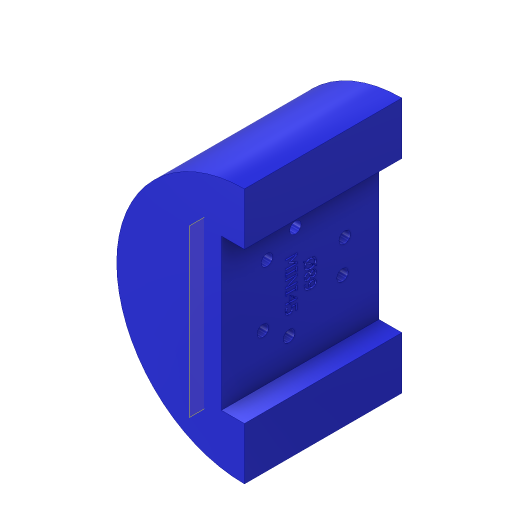
# Autodesk Inventor part: MINI45NewShell89_A
Saved by Autodesk Inventor 2023 (Build 270158000, 158)
## iProperties
Created: 2016-07-01
Part Number: MINI45NewShell89_A
Material: ABS Plastic
Document SubType Name: Modeling
Designer: Administrateur
Density: 1.06 g/cm^3
Appearance: Blue - Wall Paint - Glossy
Author: Administrateur
Autodesk Inventor part; units mm, degrees
ref_plane "XZ Plane" through (0, 0, 0) normal (0, 1, 0) x (-1, 0, 0)
sketch "Sketch1" plane through (0, 0, 0) normal (0, 0, 1) x (1, 0, 0)
  arc A0 (0, 38.9636) -> (0, -38.9636) centre (0, 0) ccw
  line L0 (0, 38.9636) -> (0, 23)
  line L1 (0, 23) -> (-7, 23)
  line L2 (-7, 23) -> (-7, 0)
  line L3 (-46.5484, 0) -> (26.4312, 0) construction
  line L4 (0, -38.9636) -> (0, -23)
  line L5 (0, -23) -> (-7, -23)
  line L6 (-7, -23) -> (-7, 0)
  dimension "d2" = 38.9636
  dimension "d3" = 46
  dimension "d4" = 7
  dimension "d27" = 23
  dimension "d28" = 15.9636
  constraints: 14 end point, 2 horizontal, 2 point on circle, 2 symmetric about line, 1 centre point, 1 coincident, 1 perpendicular, 1 vertical
  measures "d2" radius of A0
  measures "d3" distance between parallel lines of L5 L1
  measures "d4" distance of L0.end L1.end
  measures "d27" distance of L1.end L2.end
  measures "d28" distance of L0.start L0.end
extrude "Extrusion1" add sketch "Sketch1" along normal blind 48
sketch "Sketch2" plane through (-7, -23, 0) normal (1, 0, 0) x (0, 0, -1)
  line L0 (-24, 23) -> (-48, 23) construction
  line L1 (-48, 61.9636) -> (-48, -15.9636) construction
  line L2 (0, 61.9636) -> (-48, 61.9636) construction
  line L3 (-24, 61.9636) -> (-24, -15.9636) construction
  line L4 (0, -15.9636) -> (-48, -15.9636) construction
  line L5 (-24, 23) -> (-34.1427, 32.7947) construction
  circle A0 centre (-24, 23) radius 14.1 construction
  line L6 (-24, 23) -> (-25.4739, 37.0228) construction
  line L7 (-24, 23) -> (-27.4111, 9.3188) construction
  line L8 (-24, 23) -> (-35.4071, 14.7122) construction
  line L9 (-24, 23) -> (-10.4462, 26.8865) construction
  line L10 (-24, 23) -> (-11.119, 17.265) construction
  point P0 (0, 23)
  dimension "d32" = 28.2
  dimension "d34" = 40
  dimension "d37" = 360
  dimension "d39" = 84
  constraints: 16 end point, 11 coincident, 4 midpoint, 2 point on circle, 1 centre point, 17 other
  measures "d32" diameter of A0
  measures "d34" angle of L5 L6
  measures "d39" angle of L0 L6
hole "Hole1" at (-7, 14.0228, 25.4739) at (-7, 9.7947, 34.1427) at (-7, -8.2878, 35.4071) at (-7, -13.6812, 27.4111) at (-7, -5.735, 11.119) at (-7, 3.8865, 10.4462) direction (-1, 0, 0) diameter 3.5 end through all
ref_plane "Work Plane1" through (-38.9636, 0, 0) normal (1, 0, 0) x (0, 1, 0)
ref_plane "Work Plane2" through (-10, 0, 0) normal (1, 0, 0) x (0, 1, 0)
ref_plane "Work Plane3" through (-12.3, -23, 0) normal (1, 0, 0) x (0, 0, -1)
sketch "Sketch4" plane through (-12.3, -23, 0) normal (1, 0, 0) x (0, 0, -1)
  line L0 (0, 61.9636) -> (0, -15.9636) projected
  line L1 (0, -15.9636) -> (-48, -15.9636) projected
  line L2 (-48, 61.9636) -> (-48, -15.9636) projected
  line L3 (0, 61.9636) -> (-48, 61.9636) projected
  circle A0 centre (-25.4739, 37.0228) radius 1.75 projected
  circle A1 centre (-34.1427, 32.7947) radius 1.75 projected
  circle A2 centre (-35.4071, 14.7122) radius 1.75 projected
  circle A3 centre (-27.4111, 9.3188) radius 1.75 projected
  circle A4 centre (-11.119, 17.265) radius 1.75 projected
  circle A5 centre (-10.4462, 26.8865) radius 1.75 projected
  point P0 (0, 23)
  point P1 (-11.119, 19.015)
  point P2 (-35.4071, 16.4622)
  point P3 (-25.4739, 38.7728)
  point P4 (-34.1427, 34.5447)
  point P5 (-27.4111, 11.0688)
  point P6 (-10.4462, 28.6365)
  constraints: 6 coincident, 6 vertical alignment, 6 other
hole "Hole3" at (-12.3, 14.0228, 25.4739) at (-12.3, 9.7947, 34.1427) at (-12.3, -8.2878, 35.4071) at (-12.3, -13.6812, 27.4111) at (-12.3, -5.735, 11.119) at (-12.3, 3.8865, 10.4462) direction (-1, 0, 0) diameter 6.5 end through all
sketch "Sketch7" plane through (-7, -23, 0) normal (1, 0, 0) x (0, 0, -1)
  line L0 (-18.9668, 30.4561) -> (-18.9668, 14.6891) construction
  line L1 (-18.9668, 14.6891) -> (-28.3826, 14.6891) construction
  line L2 (-28.3826, 14.6891) -> (-28.3826, 30.4561) construction
  line L3 (-28.3826, 30.4561) -> (-18.9668, 30.4561) construction
  spline S0 degree 2 poles (-20.9323, 23.6518) (-21.8002, 23.6518) (-22.7561, 24.497) (-22.7561, 25.2004) knots 0 0 0 1 2 2 2
  spline S1 degree 2 poles (-22.7561, 25.2004) (-22.7561, 25.4585) (-22.6199, 25.9038) (-22.4951, 26.0825) knots 0 0 0 1 2 2 2
  line L4 (-22.4951, 26.0825) -> (-22.9546, 26.3945)
  line L5 (-22.9546, 26.3945) -> (-22.9546, 26.7405)
  line L6 (-22.9546, 26.7405) -> (-22.3023, 26.2981)
  spline S2 degree 2 poles (-22.3023, 26.2981) (-22.0697, 26.5079) (-21.3833, 26.7462) (-20.9323, 26.7462) knots 0 0 0 1 2 2 2
  spline S3 degree 2 poles (-20.9323, 26.7462) (-20.0672, 26.7462) (-19.1086, 25.8981) (-19.1086, 25.2004) knots 0 0 0 1 2 2 2
  spline S4 degree 2 poles (-19.1086, 25.2004) (-19.1086, 24.931) (-19.239, 24.5112) (-19.3667, 24.324) knots 0 0 0 1 2 2 2
  line L7 (-19.3667, 24.324) -> (-18.9668, 24.0545)
  line L8 (-18.9668, 24.0545) -> (-18.9668, 23.7057)
  line L9 (-18.9668, 23.7057) -> (-19.5567, 24.1084)
  spline S5 degree 2 poles (-19.5567, 24.1084) (-19.7893, 23.8929) (-20.4643, 23.6518) (-20.9323, 23.6518) knots 0 0 0 1 2 2 2
  spline S6 degree 2 poles (-20.9323, 24.1311) (-20.609, 24.1311) (-20.1013, 24.2616) (-19.9339, 24.3694) knots 0 0 0 1 2 2 2
  line L10 (-19.9339, 24.3694) -> (-22.1377, 25.8442)
  spline S7 degree 2 poles (-22.1377, 25.8442) (-22.2455, 25.7109) (-22.3533, 25.4103) (-22.3533, 25.1976) knots 0 0 0 1 2 2 2
  spline S8 degree 2 poles (-22.3533, 25.1976) (-22.3533, 24.7126) (-21.6215, 24.1311) (-20.9323, 24.1311) knots 0 0 0 1 2 2 2
  spline S9 degree 2 poles (-19.7212, 24.5622) (-19.6163, 24.6842) (-19.5113, 25.0047) (-19.5113, 25.1976) knots 0 0 0 1 2 2 2
  spline S10 degree 2 poles (-19.5113, 25.1976) (-19.5113, 25.6854) (-20.2346, 26.2669) (-20.9323, 26.2669) knots 0 0 0 1 2 2 2
  spline S11 degree 2 poles (-20.9323, 26.2669) (-21.25, 26.2669) (-21.7435, 26.1449) (-21.9193, 26.0343) knots 0 0 0 1 2 2 2
  line L11 (-21.9193, 26.0343) -> (-19.7212, 24.5622)
  spline S12 degree 2 poles (-22.7617, 22.1826) (-22.7617, 22.4435) (-22.6057, 22.8718) (-22.4611, 23.0221) knots 0 0 0 1 2 2 2
  spline S13 degree 2 poles (-22.4611, 23.0221) (-22.3193, 23.1696) (-21.9335, 23.3228) (-21.7151, 23.3228) knots 0 0 0 1 2 2 2
  spline S14 degree 2 poles (-21.7151, 23.3228) (-21.4315, 23.3228) (-20.955, 23.0193) (-20.8132, 22.73) knots 0 0 0 1 2 2 2
  line L12 (-20.8132, 22.73) -> (-20.799, 22.73)
  spline S15 degree 2 poles (-20.799, 22.73) (-20.6487, 22.9881) (-20.2913, 23.2377) (-20.0247, 23.2377) knots 0 0 0 1 2 2 2
  spline S16 degree 2 poles (-20.0247, 23.2377) (-19.6305, 23.2377) (-19.1029, 22.6421) (-19.1029, 22.1826) knots 0 0 0 1 2 2 2
  spline S17 degree 2 poles (-19.1029, 22.1826) (-19.1029, 21.7061) (-19.6021, 21.1303) (-19.9935, 21.1303) knots 0 0 0 1 2 2 2
  spline S18 degree 2 poles (-19.9935, 21.1303) (-20.2289, 21.1303) (-20.6884, 21.4054) (-20.8189, 21.6635) knots 0 0 0 1 2 2 2
  line L13 (-20.8189, 21.6635) -> (-20.833, 21.6635)
  spline S19 degree 2 poles (-20.833, 21.6635) (-20.9749, 21.3572) (-21.3833, 21.0424) (-21.7066, 21.0424) knots 0 0 0 1 2 2 2
  spline S20 degree 2 poles (-21.7066, 21.0424) (-22.1548, 21.0424) (-22.7617, 21.6947) (-22.7617, 22.1826) knots 0 0 0 1 2 2 2
  spline S21 degree 2 poles (-21.752, 21.5246) (-21.5364, 21.5246) (-21.2812, 21.6947) (-21.1507, 21.9358) knots 0 0 0 1 2 2 2
  spline S22 degree 2 poles (-21.1507, 21.9358) (-21.1053, 22.0152) (-21.0004, 22.2818) (-20.9323, 22.4492) knots 0 0 0 1 2 2 2
  spline S23 degree 2 poles (-20.9323, 22.4492) (-21.0599, 22.6421) (-21.44, 22.8491) (-21.6811, 22.8491) knots 0 0 0 1 2 2 2
  spline S24 degree 2 poles (-21.6811, 22.8491) (-21.9988, 22.8491) (-22.4129, 22.4662) (-22.4129, 22.1769) knots 0 0 0 1 2 2 2
  spline S25 degree 2 poles (-22.4129, 22.1769) (-22.4129, 21.8819) (-22.0583, 21.5246) (-21.752, 21.5246) knots 0 0 0 1 2 2 2
  spline S26 degree 2 poles (-19.9992, 21.5898) (-19.7638, 21.5898) (-19.4489, 21.9046) (-19.4489, 22.1854) knots 0 0 0 1 2 2 2
  spline S27 degree 2 poles (-19.4489, 22.1854) (-19.4489, 22.4407) (-19.7297, 22.7669) (-19.9708, 22.7669) knots 0 0 0 1 2 2 2
  spline S28 degree 2 poles (-19.9708, 22.7669) (-20.1438, 22.7669) (-20.3849, 22.5995) (-20.4813, 22.4322) knots 0 0 0 1 2 2 2
  spline S29 degree 2 poles (-20.4813, 22.4322) (-20.5211, 22.3613) (-20.66, 22.0606) (-20.6997, 21.9387) knots 0 0 0 1 2 2 2
  spline S30 degree 2 poles (-20.6997, 21.9387) (-20.5437, 21.7344) (-20.2119, 21.5898) (-19.9992, 21.5898) knots 0 0 0 1 2 2 2
  spline S31 degree 2 poles (-20.3197, 20.7105) (-20.0502, 20.7105) (-19.6021, 20.5347) (-19.4404, 20.3815) knots 0 0 0 1 2 2 2
  spline S32 degree 2 poles (-19.4404, 20.3815) (-19.2844, 20.2369) (-19.1114, 19.8143) (-19.1114, 19.5987) knots 0 0 0 1 2 2 2
  spline S33 degree 2 poles (-19.1114, 19.5987) (-19.1114, 19.3576) (-19.2731, 18.9662) (-19.4262, 18.8216) knots 0 0 0 1 2 2 2
  spline S34 degree 2 poles (-19.4262, 18.8216) (-19.6191, 18.64) (-20.2431, 18.4415) (-20.7224, 18.4415) knots 0 0 0 1 2 2 2
  spline S35 degree 2 poles (-20.7224, 18.4415) (-21.1564, 18.4415) (-21.9335, 18.6372) (-22.1916, 18.8272) knots 0 0 0 1 2 2 2
  spline S36 degree 2 poles (-22.1916, 18.8272) (-22.4639, 19.0286) (-22.7504, 19.5959) (-22.7504, 20.01) knots 0 0 0 1 2 2 2
  spline S37 degree 2 poles (-22.7504, 20.01) (-22.7504, 20.1036) (-22.7305, 20.3163) (-22.7022, 20.407) knots 0 0 0 1 2 2 2
  line L14 (-22.7022, 20.407) -> (-22.2512, 20.407)
  line L15 (-22.2512, 20.407) -> (-22.2512, 20.3844)
  spline S38 degree 2 poles (-22.2512, 20.3844) (-22.2852, 20.3248) (-22.3448, 20.0752) (-22.3448, 19.9476) knots 0 0 0 1 2 2 2
  spline S39 degree 2 poles (-22.3448, 19.9476) (-22.3448, 19.4881) (-21.7378, 18.9634) (-21.1762, 18.9265) knots 0 0 0 1 2 2 2
  spline S40 degree 2 poles (-21.1762, 18.9265) (-21.3039, 19.1137) (-21.4202, 19.454) (-21.4202, 19.6554) knots 0 0 0 1 2 2 2
  spline S41 degree 2 poles (-21.4202, 19.6554) (-21.4202, 19.8483) (-21.3351, 20.1688) (-21.2131, 20.3305) knots 0 0 0 1 2 2 2
  spline S42 degree 2 poles (-21.2131, 20.3305) (-21.0685, 20.5177) (-20.6288, 20.7105) (-20.3197, 20.7105) knots 0 0 0 1 2 2 2
  spline S43 degree 2 poles (-20.6175, 18.9152) (-20.2629, 18.9152) (-19.8148, 19.0456) (-19.6928, 19.1619) knots 0 0 0 1 2 2 2
  spline S44 degree 2 poles (-19.6928, 19.1619) (-19.5794, 19.264) (-19.4943, 19.4767) (-19.4943, 19.6015) knots 0 0 0 1 2 2 2
  spline S45 degree 2 poles (-19.4943, 19.6015) (-19.4943, 19.8908) (-19.9084, 20.234) (-20.2998, 20.234) knots 0 0 0 1 2 2 2
  spline S46 degree 2 poles (-20.2998, 20.234) (-20.5211, 20.234) (-20.8075, 20.1206) (-20.9096, 19.9958) knots 0 0 0 1 2 2 2
  spline S47 degree 2 poles (-20.9096, 19.9958) (-20.9834, 19.905) (-21.0316, 19.681) (-21.0316, 19.5505) knots 0 0 0 1 2 2 2
  spline S48 degree 2 poles (-21.0316, 19.5505) (-21.0316, 19.4002) (-20.9266, 19.0541) (-20.8387, 18.9237) knots 0 0 0 1 2 2 2
  spline S49 degree 2 poles (-20.8387, 18.9237) (-20.8047, 18.9208) (-20.6884, 18.9152) (-20.6175, 18.9152) knots 0 0 0 1 2 2 2
  line L16 (-28.445, 27.1007) -> (-28.445, 27.5659)
  line L17 (-28.445, 27.5659) -> (-25.43, 27.5659)
  line L18 (-25.43, 27.5659) -> (-27.4806, 28.4792)
  line L19 (-27.4806, 28.4792) -> (-27.4806, 28.7628)
  line L20 (-27.4806, 28.7628) -> (-25.43, 29.6676)
  line L21 (-25.43, 29.6676) -> (-28.445, 29.6676)
  line L22 (-28.445, 29.6676) -> (-28.445, 30.1015)
  line L23 (-28.445, 30.1015) -> (-24.945, 30.1015)
  line L24 (-24.945, 30.1015) -> (-24.945, 29.4662)
  line L25 (-24.945, 29.4662) -> (-26.8935, 28.5926)
  line L26 (-26.8935, 28.5926) -> (-24.945, 27.7474)
  line L27 (-24.945, 27.7474) -> (-24.945, 27.1007)
  line L28 (-24.945, 27.1007) -> (-28.445, 27.1007)
  line L29 (-28.445, 25.172) -> (-28.445, 26.5278)
  line L30 (-28.445, 26.5278) -> (-28.0876, 26.5278)
  line L31 (-28.0876, 26.5278) -> (-28.0876, 26.0825)
  line L32 (-28.0876, 26.0825) -> (-25.3023, 26.0825)
  line L33 (-25.3023, 26.0825) -> (-25.3023, 26.5278)
  line L34 (-25.3023, 26.5278) -> (-24.945, 26.5278)
  line L35 (-24.945, 26.5278) -> (-24.945, 25.172)
  line L36 (-24.945, 25.172) -> (-25.3023, 25.172)
  line L37 (-25.3023, 25.172) -> (-25.3023, 25.6173)
  line L38 (-25.3023, 25.6173) -> (-28.0876, 25.6173)
  line L39 (-28.0876, 25.6173) -> (-28.0876, 25.172)
  line L40 (-28.0876, 25.172) -> (-28.445, 25.172)
  line L41 (-28.445, 22.0918) -> (-28.445, 22.6137)
  line L42 (-28.445, 22.6137) -> (-25.4271, 24.1623)
  line L43 (-25.4271, 24.1623) -> (-28.445, 24.1623)
  line L44 (-28.445, 24.1623) -> (-28.445, 24.5963)
  line L45 (-28.445, 24.5963) -> (-24.945, 24.5963)
  line L46 (-24.945, 24.5963) -> (-24.945, 23.9354)
  line L47 (-24.945, 23.9354) -> (-27.716, 22.5258)
  line L48 (-27.716, 22.5258) -> (-24.945, 22.5258)
  line L49 (-24.945, 22.5258) -> (-24.945, 22.0918)
  line L50 (-24.945, 22.0918) -> (-28.445, 22.0918)
  line L51 (-28.445, 20.1631) -> (-28.445, 21.5189)
  line L52 (-28.445, 21.5189) -> (-28.0876, 21.5189)
  line L53 (-28.0876, 21.5189) -> (-28.0876, 21.0736)
  line L54 (-28.0876, 21.0736) -> (-25.3023, 21.0736)
  line L55 (-25.3023, 21.0736) -> (-25.3023, 21.5189)
  line L56 (-25.3023, 21.5189) -> (-24.945, 21.5189)
  line L57 (-24.945, 21.5189) -> (-24.945, 20.1631)
  line L58 (-24.945, 20.1631) -> (-25.3023, 20.1631)
  line L59 (-25.3023, 20.1631) -> (-25.3023, 20.6084)
  line L60 (-25.3023, 20.6084) -> (-28.0876, 20.6084)
  line L61 (-28.0876, 20.6084) -> (-28.0876, 20.1631)
  line L62 (-28.0876, 20.1631) -> (-28.445, 20.1631)
  line L63 (-27.2424, 17.4346) -> (-27.2424, 17.8515)
  line L64 (-27.2424, 17.8515) -> (-28.445, 17.8515)
  line L65 (-28.445, 17.8515) -> (-28.445, 18.3025)
  line L66 (-28.445, 18.3025) -> (-27.2424, 18.3025)
  line L67 (-27.2424, 18.3025) -> (-27.2424, 19.8483)
  line L68 (-27.2424, 19.8483) -> (-26.7489, 19.8483)
  line L69 (-26.7489, 19.8483) -> (-24.945, 18.2827)
  line L70 (-24.945, 18.2827) -> (-24.945, 17.8515)
  line L71 (-24.945, 17.8515) -> (-26.8652, 17.8515)
  line L72 (-26.8652, 17.8515) -> (-26.8652, 17.4346)
  line L73 (-26.8652, 17.4346) -> (-27.2424, 17.4346)
  line L74 (-26.8652, 18.3025) -> (-25.4981, 18.3025)
  line L75 (-25.4981, 18.3025) -> (-26.8652, 19.4796)
  line L76 (-26.8652, 19.4796) -> (-26.8652, 18.3025)
  spline S50 degree 2 poles (-27.3331, 14.9387) (-27.5856, 14.9387) (-28.0167, 15.1003) (-28.1755, 15.2478) knots 0 0 0 1 2 2 2
  spline S51 degree 2 poles (-28.1755, 15.2478) (-28.3344, 15.3953) (-28.5187, 15.8349) (-28.5187, 16.1072) knots 0 0 0 1 2 2 2
  spline S52 degree 2 poles (-28.5187, 16.1072) (-28.5187, 16.3568) (-28.4081, 16.8446) (-28.3202, 17.0233) knots 0 0 0 1 2 2 2
  line L77 (-28.3202, 17.0233) -> (-27.8238, 17.0233)
  line L78 (-27.8238, 17.0233) -> (-27.8238, 16.9893)
  spline S53 degree 2 poles (-27.8238, 16.9893) (-27.8635, 16.9354) (-27.9656, 16.734) (-28.011, 16.6121) knots 0 0 0 1 2 2 2
  spline S54 degree 2 poles (-28.011, 16.6121) (-28.0592, 16.4731) (-28.1131, 16.2434) (-28.1131, 16.0987) knots 0 0 0 1 2 2 2
  spline S55 degree 2 poles (-28.1131, 16.0987) (-28.1131, 15.9569) (-28.011, 15.6903) (-27.9004, 15.5938) knots 0 0 0 1 2 2 2
  spline S56 degree 2 poles (-27.9004, 15.5938) (-27.7955, 15.5059) (-27.5175, 15.4152) (-27.3303, 15.4152) knots 0 0 0 1 2 2 2
  spline S57 degree 2 poles (-27.3303, 15.4152) (-27.1431, 15.4152) (-26.9049, 15.5173) (-26.8254, 15.6137) knots 0 0 0 1 2 2 2
  spline S58 degree 2 poles (-26.8254, 15.6137) (-26.7375, 15.713) (-26.6638, 16.0079) (-26.6638, 16.1866) knots 0 0 0 1 2 2 2
  spline S59 degree 2 poles (-26.6638, 16.1866) (-26.6638, 16.3795) (-26.7233, 16.7624) (-26.7489, 16.8787) knots 0 0 0 1 2 2 2
  line L79 (-26.7489, 16.8787) -> (-24.945, 16.8787)
  line L80 (-24.945, 16.8787) -> (-24.945, 14.9585)
  line L81 (-24.945, 14.9585) -> (-25.3562, 14.9585)
  line L82 (-25.3562, 14.9585) -> (-25.3562, 16.4277)
  line L83 (-25.3562, 16.4277) -> (-26.2894, 16.4277)
  spline S60 degree 2 poles (-26.2894, 16.4277) (-26.278, 16.3426) (-26.2695, 16.1781) (-26.2695, 16.11) knots 0 0 0 1 2 2 2
  spline S61 degree 2 poles (-26.2695, 16.11) (-26.2695, 15.8406) (-26.3575, 15.469) (-26.4879, 15.2989) knots 0 0 0 1 2 2 2
  spline S62 degree 2 poles (-26.4879, 15.2989) (-26.6184, 15.1258) (-27.0155, 14.9387) (-27.3331, 14.9387) knots 0 0 0 1 2 2 2
  point P0 (0, 23)
  constraints: 2 other
extrude "Extrusion3" cut sketch "Sketch7" against normal blind 1
equation "\"d27\" = 0.5 * d3"
equation "\"d28\" = -0.5 * d3 + d2"
body "Solid1"
